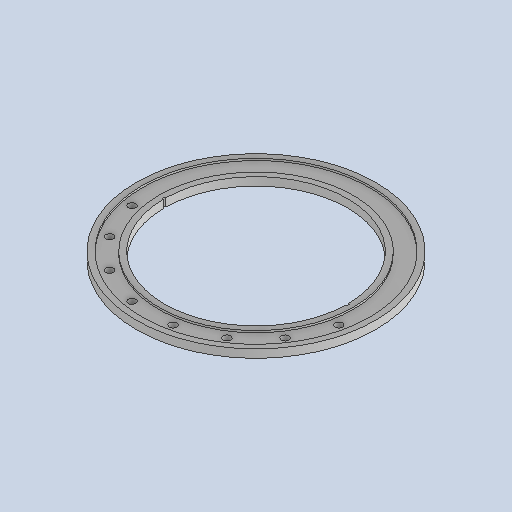
# Autodesk Inventor part: ДМФ 021 кольцо прижимное нос
Saved by Autodesk Inventor 2025 (Build 290162010, 162A)
## iProperties
Created: 2024-04-23
Part Number: ДМФ 021 кольцо прижимное нос
Material: Generic
Document SubType Name: Sheet Metal
Designer: admin
Density: 1 g/cm^3
Appearance: Default
Flat Pattern Width: 44.2 cm
Flat Pattern Length: 44.2 cm
Flat Pattern Area: 1953.64 cm^2
Sheet Metal Rule: Default
Sheet Metal Width: 442,000 mm
Sheet Metal Length: 442,000 mm
Sheet Metal Area: 195364,000 mm^2
Author: admin
Autodesk Inventor part; units mm, degrees
note: some values were not read from the file. Chosen so that the rebuilt part matches the saved one: pattern direction of "Circular Pattern2".
ref_plane "YZ Plane" through (0, 0, 0) normal (1, 0, 0) x (0, 1, 0)
ref_plane "XZ Plane" through (0, 0, 0) normal (0, 1, 0) x (-1, 0, 0)
ref_plane "XY Plane" through (0, 0, 0) normal (0, 0, 1) x (1, 0, 0)
sketch "Sketch1" plane through (0, 0, 0) normal (0, 0, 1) x (1, 0, 0)
  circle A0 centre (0, 0) radius 169
  circle A1 centre (0, 0) radius 221
  circle A2 centre (0, 0) radius 195 construction
  line L0 (0, 169) -> (0, 221) construction
  point P0 (0, 195)
  dimension "d17" = 390
  dimension "d18" = 52
  constraints: 4 vertical alignment, 3 coincident, 2 end point, 1 midpoint, 1 vertical, 6 other
  measures "d18" distance of L0.start L0.end
extrude "Extrusion1" add sketch "Sketch1" along normal blind 15
sketch "Sketch2" plane through (0, 0, 15) normal (0, 0, 1) x (1, 0, 0)
  circle A0 centre (0, 0) radius 221 construction
  circle A1 centre (0, 0) radius 169 construction
  line L0 (0, 210.5) -> (0, 179.5) construction
  line L1 (0, 169) -> (0, 0) construction
  circle A2 centre (0, 0) radius 179.5
  circle A3 centre (0, 0) radius 210.5
  circle A4 centre (0, 0) radius 195 construction
  point P0 (0, 195)
  dimension "d19" = 390
  dimension "d4" = 31
  constraints: 5 vertical alignment, 4 end point, 3 coincident, 2 vertical, 1 midpoint, 7 other
  measures "d4" distance of L0.start L0.end
extrude "Extrusion2" cut sketch "Sketch2" against normal blind 3.5
sketch "Sketch3" plane through (0, 0, 0) normal (0, 0, 1) x (1, 0, 0)
  circle A0 centre (0, 0) radius 169 construction
  circle A1 centre (0, 0) radius 221 construction
  circle A2 centre (0, 0) radius 179.5 projected
  circle A3 centre (0, 0) radius 210.5 projected
  circle A4 centre (0, 0) radius 221 projected
  line L0 (0, 0) -> (0, -221) construction
  line L1 (0, 0) -> (43.115, -216.7535) construction
  line L2 (35.0187, -176.051) -> (41.0665, -206.4553) construction
  circle A5 centre (38.0426, -191.2531) radius 7
  dimension "d20" = 11.25
  dimension "d21" = 14
  constraints: 6 end point, 2 point on circle, 2 point on line, 1 centre point, 1 midpoint, 1 vertical, 4 other
  measures "d20" angle of L1 L0
  measures "d21" diameter of A5
extrude "Extrusion3" cut sketch "Sketch3" along normal through all contours A5
pattern_circular "Circular Pattern2" count 8 over 157.5 about axis through (0, 0, 0) along (0, 0, -1) of "Extrusion3" both ways yes
sketch "Sketch5" plane through (0, 0, 0) normal (0, 0, -1) x (-1, 0, 0)
  circle A0 centre (0, 0) radius 169 projected
  circle A1 centre (0, 0) radius 221 projected
  line L0 (0, 0) -> (169, 0) construction
  arc A2 (168.9815, -2.4999) -> (168.9815, 2.4999) centre (169, 0) ccw
  dimension "d36" = 5
  constraints: 5 point on circle, 2 end point, 1 centre point, 1 coincident, 1 horizontal
  measures "d36" diameter of A2
extrude "Extrusion4" cut sketch "Sketch5" against normal through all contours A0 A2
mirror "Mirror1" about plane through (0, 0, 0) normal (1, 0, 0) of "Extrusion4"
equation "\"d17\" = Шпил_пласт_НОС_диам_центров"
equation "\"d19\" = Шпил_пласт_НОС_диам_центров"
equation "\"BendReliefDepth\" = 0.5 * Thickness"
equation "\"Шпил_пласт_НОС_диам_центров\" = 390"
equation "\"Thickness\" = 10"
body "Solid1"
